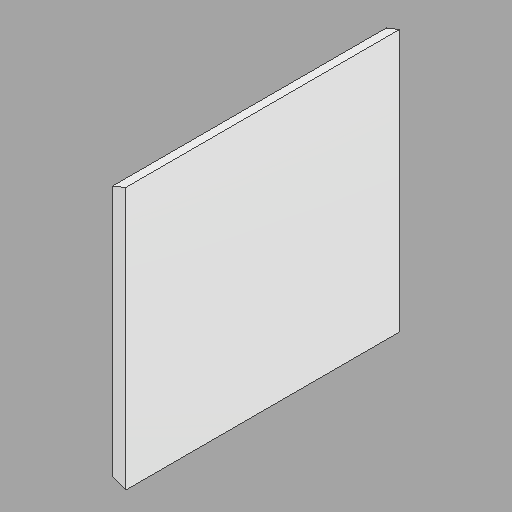
# Autodesk Inventor part: door2
Saved by Autodesk Inventor 2025.2 (Build 292293000, 293)
## iProperties
Created: 2025-02-23
Part Number: door2
Material: ABS Plastic
Document SubType Name: Modeling
Designer: Alex
Density: 1.06 g/cm^3
Appearance: Smooth - White
Author: Alex
Autodesk Inventor part; units mm, degrees
ref_plane "YZ Plane" through (0, 0, 0) normal (1, 0, 0) x (0, 1, 0)
ref_plane "XZ Plane" through (0, 0, 0) normal (0, 1, 0) x (-1, 0, 0)
ref_plane "XY Plane" through (0, 0, 0) normal (0, 0, 1) x (1, 0, 0)
sketch "Sketch1" plane through (0, 0, 0) normal (0, 0, 1) x (1, 0, 0)
  line L0 (44.8, 3.5) -> (44.8, 89.5) construction
  line L1 (-45, 89.5) -> (44.8, 89.5) construction
  line L2 (-45, 94.5) -> (-45, 89.5) construction
  line L3 (-50, 92.5) -> (-45, 94.5) construction
  line L4 (-50, 0.5) -> (-50, 92.5) construction
  line L5 (-45, -1.5) -> (-50, 0.5) construction
  line L6 (-45, 3.5) -> (-45, -1.5) construction
  line L7 (44.8, 3.5) -> (-45, 3.5) construction
  line L8 (-49.9, 92.4323) -> (-45.1, 94.3523)
  line L9 (-45.1, 94.3523) -> (-45.1, 89.4)
  line L10 (-45.1, 89.4) -> (44.7, 89.4) construction
  line L11 (44.7, 89.4) -> (44.7, 3.6) construction
  line L12 (44.7, 3.6) -> (-45.1, 3.6) construction
  line L13 (-45.1, 3.6) -> (-45.1, -1.3523)
  line L14 (-45.1, -1.3523) -> (-49.9, 0.5677)
  line L15 (-49.9, 0.5677) -> (-49.9, 92.4323)
  line L16 (-45.1, 89.4) -> (-45.1, 3.6)
  point P0 (0, 0)
  dimension "d0" = 0.1
  constraints: 18 end point, 1 collinear, 7 other
  measures "d0" distance between parallel lines of L4 L15
extrude "Extrusion1" add sketch "Sketch1" against normal blind 100
sketch "Sketch2" plane through (-49.9, 0.5677, -100) normal (-0.3713907, -0.9284767, 0) x (0.9284767, -0.3713907, 0)
  circle A0 centre (2.5849, 10) radius 1
  line L0 (5.1698, 0) -> (0, 0) projected
  line L1 (2.5849, 0) -> (2.5849, 10) construction
  point P0 (46.5418, 100)
  dimension "d3" = 2
  dimension "d4" = 10
  constraints: 2 end point, 1 centre point, 1 midpoint, 1 vertical
  measures "d3" diameter of A0
  measures "d4" distance of L1.start L1.end
extrude "Extrusion2" add sketch "Sketch2" along normal blind 0.7
fillet "Fillet1" radius 1 2 edges at (-48.6885, -0.6708, -90) (-48.4285, -0.0209, -90)
body "Solid1"
